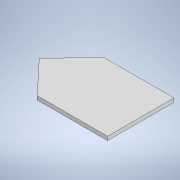
# Autodesk Inventor part: lidar_base
Saved by Autodesk Inventor 2022 (Build 260153000, 153)
## iProperties
Created: 2022-08-18
Part Number: lidar_base
Material: Generic
Document SubType Name: Modeling
Designer: Alok
Density: 1 g/cm^3
Appearance: Default
Author: Alok
Autodesk Inventor part; units mm, degrees
ref_plane "YZ Plane" through (0, 0, 0) normal (1, 0, 0) x (0, 1, 0)
ref_plane "XZ Plane" through (0, 0, 0) normal (0, 1, 0) x (-1, 0, 0)
ref_plane "XY Plane" through (0, 0, 0) normal (0, 0, 1) x (1, 0, 0)
sketch "Sketch1" plane through (0, 0, 0) normal (0, 1, 0) x (-1, 0, 0)
  line L0 (45, 42.5) -> (-45, 42.5)
  line L1 (-45, 42.5) -> (-45, -42.5)
  line L2 (-45, -42.5) -> (45, -42.5)
  line L3 (45, 42.5) -> (-45, -42.5) construction
  line L4 (-45, 42.5) -> (45, -42.5) construction
  line L5 (45, 42.5) -> (85, 0)
  line L6 (85, 0) -> (45, -42.5)
  point P0 (0, 0)
  dimension "d0" = 90
  dimension "d1" = 85
  constraints: 14 end point, 2 midpoint, 1 horizontal, 1 parallel, 1 perpendicular
  measures "d0" distance of L2.end L1.end
  measures "d1" distance of L1.end L0.end
extrude "Extrusion1" add sketch "Sketch1" along normal blind 5
body "Solid1"
